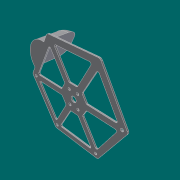
# Autodesk Inventor part: CoilCover
Saved by Autodesk Inventor 2020.4 (Build 244396010, 396A)
## iProperties
Created: 2022-09-10
Part Number: CoilCover
Material: Generic
Document SubType Name: Sheet Metal
Designer: Val
Density: 1 g/cm^3
Sheet Metal Rule: Default
Appearance: Default
Author: Val
Autodesk Inventor part; units mm, degrees
ref_plane "YZ Plane" through (0, 0, 0) normal (1, 0, 0) x (0, 1, 0)
ref_plane "XZ Plane" through (0, 0, 0) normal (0, 1, 0) x (-1, 0, 0)
ref_plane "XY Plane" through (0, 0, 0) normal (0, 0, 1) x (1, 0, 0)
sketch "Base" plane through (0, 0, 0) normal (0, 0, 1) x (1, 0, 0)
  arc A0 (-112.5402, 3.048) -> (-112.5402, -3.048) centre (-107.2609, 0) ccw
  line L0 (-58.9098, 95.9387) -> (-112.5402, 3.048)
  line L1 (-112.5402, -3.048) -> (-58.9098, -95.9387)
  arc A1 (-58.9098, -95.9387) -> (-53.6305, -98.9867) centre (-53.6305, -92.8907) ccw
  arc A2 (53.6305, -98.9867) -> (58.9098, -95.9387) centre (53.6305, -92.8907) ccw
  arc A3 (112.5402, -3.048) -> (112.5402, 3.048) centre (107.2609, 0) ccw
  arc A4 (58.9098, 95.9387) -> (53.6305, 98.9867) centre (53.6305, 92.8907) ccw
  arc A5 (-53.6305, 98.9867) -> (-58.9098, 95.9387) centre (-53.6305, 92.8907) ccw
  line L2 (-53.6305, 98.9867) -> (53.6305, 98.9867)
  line L3 (112.5402, 3.048) -> (58.9098, 95.9387)
  line L4 (58.9098, 95.9387) -> (112.5402, 3.048)
  arc A6 (53.6305, -98.9867) -> (58.9098, -95.9387) centre (53.6305, -92.8907) ccw
  line L5 (112.5402, -3.048) -> (58.9098, -95.9387)
  line L6 (-53.6305, -98.9867) -> (53.6305, -98.9867)
  line L7 (0, 98.9867) -> (0, -98.9867) construction
  line L8 (-113.3569, 0) -> (113.3569, 0) construction
  point P0 (0, 0)
  point P1 (0, 0)
  dimension "d0" = 6.096
  dimension "d1" = 107.2609
  dimension "d2" = 120
  dimension "d3" = 120
  dimension "d4" = 120
  dimension "d5" = 120
  dimension "d6" = 120
  measures "d0" radius of A4
  measures "d1" distance of L2.start L2.end
  measures "d2" angle of L2 L0
  measures "d3" angle of L3 L2
  measures "d4" angle of L6 L1
  measures "d5" angle of L5 L6
  measures "d6" angle of L1 L0
extrude "Plate1" add sketch "Base" along normal blind 3.048
sketch "Cuts" plane through (0, 0, 0) normal (0, 0, -1) x (-1, 0, 0)
  line L0 (0, 0) -> (-56.6785, 98.17) construction
  line L1 (0, 0) -> (-113.3569, 0) construction
  line L2 (0, 0) -> (-56.6785, -98.17) construction
  arc A0 (-53.6305, 98.9867) -> (-58.9098, 95.9387) centre (-53.6305, 92.8907) ccw projected
  arc A1 (-112.5402, 3.048) -> (-112.5402, -3.048) centre (-107.2609, 0) ccw projected
  arc A2 (-58.9098, -95.9387) -> (-53.6305, -98.9867) centre (-53.6305, -92.8907) ccw projected
  line L3 (-112.5402, 3.048) -> (-58.9098, 95.9387) projected
  line L4 (-95.9691, 6.35) -> (-53.4838, 79.9367)
  line L5 (-53.4838, 79.9367) -> (-10.9985, 6.35)
  line L6 (-10.9985, 6.35) -> (-95.9691, 6.35)
  line L7 (-95.9691, -6.35) -> (-53.4838, -79.9367)
  line L8 (-53.4838, -79.9367) -> (-10.9985, -6.35)
  line L9 (-10.9985, -6.35) -> (-95.9691, -6.35)
  line L10 (0, 0) -> (56.6785, 98.17) construction
  arc A3 (58.9098, 95.9387) -> (53.6305, 98.9867) centre (53.6305, 92.8907) ccw projected
  line L11 (0, 0) -> (56.6785, -98.17) construction
  arc A4 (53.6305, -98.9867) -> (58.9098, -95.9387) centre (53.6305, -92.8907) ccw projected
  line L12 (-42.4853, 86.2867) -> (42.4853, 86.2867)
  line L13 (42.4853, 86.2867) -> (0, 12.7)
  line L14 (0, 12.7) -> (-42.4853, 86.2867)
  line L15 (-53.6305, 98.9867) -> (53.6305, 98.9867) projected
  line L16 (-42.4853, -86.2867) -> (42.4853, -86.2867)
  line L17 (42.4853, -86.2867) -> (0, -12.7)
  line L18 (0, -12.7) -> (-42.4853, -86.2867)
  line L19 (0, 0) -> (0, 98.9867) construction
  line L20 (53.6305, 98.9867) -> (-53.6305, 98.9867) projected
  line L21 (95.9691, 6.35) -> (53.4838, 79.9367)
  line L22 (53.4838, 79.9367) -> (10.9985, 6.35)
  line L23 (10.9985, 6.35) -> (95.9691, 6.35)
  line L24 (95.9691, -6.35) -> (53.4838, -79.9367)
  line L25 (53.4838, -79.9367) -> (10.9985, -6.35)
  line L26 (10.9985, -6.35) -> (95.9691, -6.35)
  circle A5 centre (0, 0) radius 6.35
  circle A6 centre (51.5968, 89.3682) radius 3.175
  line L27 (58.9098, 95.9387) -> (112.5402, 3.048) projected
  circle A7 centre (51.5968, 89.3682) radius 9.6185 construction
  arc A8 (112.5402, -3.048) -> (112.5402, 3.048) centre (107.2609, 0) ccw projected
  line L28 (113.3569, 0) -> (0, 0) construction
  circle A9 centre (103.1936, 0) radius 9.6185 construction
  line L29 (112.5402, -3.048) -> (58.9098, -95.9387) projected
  circle A10 centre (103.1936, 0) radius 3.175
  circle A11 centre (51.5968, -89.3682) radius 9.6185 construction
  line L30 (53.6305, -98.9867) -> (-53.6305, -98.9867) projected
  circle A12 centre (51.5968, -89.3682) radius 3.175
  circle A13 centre (-51.5968, 89.3682) radius 3.175
  circle A14 centre (-103.1936, 0) radius 3.175
  circle A15 centre (-51.5968, -89.3682) radius 3.175
  dimension "d12" = 12.7
  dimension "d13" = 6.35
  dimension "d14" = 6.35
  dimension "d15" = 12.7
  dimension "d16" = 6.35
  dimension "d17" = 6.35
  dimension "d21" = 12.7
  dimension "d22" = 6.35
  dimension "d24" = 6.35
  dimension "d25" = 6.35
  constraints: 50 end point, 15 symmetric about line, 8 centre point, 8 point on circle, 5 parallel, 4 coincident, 3 horizontal, 3 point on line, 1 midpoint, 1 tangent, 11 other
  measures "d12" distance between parallel lines of L3 L4
  measures "d13" distance between parallel lines of L0 L5
  measures "d14" distance between parallel lines of L1 L6
  measures "d15" distance between parallel lines of L15 L12
  measures "d16" distance between parallel lines of L0 L14
  measures "d17" distance between parallel lines of L10 L13
  measures "d21" diameter of A5
  measures "d22" diameter of A6
  measures "d24" diameter of A10
  measures "d25" diameter of A12
extrude "CutsFeature" cut sketch "Cuts" against normal blind 3.048 contours L4 L5 L6 | L9 L8 L7 | L12 L13 L14 | L18 L17 L16 | L23 L22 L21 | L24 L25 L26 | A5 | A10 | A12 | A14 | A15
chamfer "Corner Chamfer1" distance 19.05 angle 45 6 edges at (-10.9985, 6.35, 1.524) (0, 12.7, 1.524) (10.9985, 6.35, 1.524) (10.9985, -6.35, 1.524) (0, -12.7, 1.524) (-10.9985, -6.35, 1.524)
fillet "InsideFilletsFeature" radius 3.175 24 edges at (-42.4853, 86.2867, 1.524) (-53.4838, 79.9367, 1.524) (-95.9691, 6.35, 1.524) (42.4853, 86.2867, 1.524) (-53.4838, -79.9367, 1.524) (-95.9691, -6.35, 1.524) (-42.4853, -86.2867, 1.524) (42.4853, -86.2867, 1.524) (53.4838, -79.9367, 1.524) (95.9691, -6.35, 1.524) (95.9691, 6.35, 1.524) (53.4838, 79.9367, 1.524) (30.0485, -6.35, 1.524) (20.5235, -22.8478, 1.524) (30.0485, 6.35, 1.524) (20.5235, 22.8478, 1.524) (9.525, 29.1978, 1.524) (-9.525, 29.1978, 1.524) (-20.5235, 22.8478, 1.524) (-30.0485, 6.35, 1.524) (-30.0485, -6.35, 1.524) (-20.5235, -22.8478, 1.524) (-9.525, -29.1978, 1.524) (9.525, -29.1978, 1.524)
sketch "Sketch4" plane through (0, 0, 0) normal (0, 0, -1) x (-1, 0, 0)
  circle A0 centre (10, 16) radius 3 projected
  circle A1 centre (-10, 16) radius 3 projected
  circle A2 centre (10, -16) radius 3 projected
  circle A3 centre (-10, -16) radius 3 projected
  point P0 (0, 0)
extrude "Cut2" cut sketch "Sketch4" against normal blind 3.048
sketch "Sketch5" plane through (0, 0, 0) normal (0, 0, -1) x (-1, 0, 0)
  circle A0 centre (-10, 16) radius 3 projected
  circle A1 centre (0, 0) radius 18.868 construction
  circle A2 centre (0, 0) radius 11.43 construction
  circle A3 centre (0, 0) radius 25.4 construction
  line L0 (-19.7973, 11.43) -> (-12.0984, 6.985) construction
  line L1 (-21.0673, 9.2303) -> (-13.3684, 4.7853)
  line L2 (-10.8284, 9.1847) -> (-18.5273, 13.6297)
  arc A4 (-18.5273, 13.6297) -> (-21.0673, 9.2303) centre (-19.7973, 11.43) ccw
  arc A5 (-13.3684, 4.7853) -> (-10.8284, 9.1847) centre (-12.0984, 6.985) ccw
  circle A6 centre (0, 0) radius 6.35 construction
  line L3 (-13.97, 2.54) -> (-22.86, 2.54)
  arc A7 (-22.86, 2.54) -> (-22.86, -2.54) centre (-22.86, 0) ccw
  line L4 (-22.86, -2.54) -> (-13.97, -2.54)
  arc A8 (-13.97, -2.54) -> (-13.97, 2.54) centre (-13.97, 0) ccw
  line L5 (-13.3684, -4.7853) -> (-21.0673, -9.2303)
  arc A9 (-21.0673, -9.2303) -> (-18.5273, -13.6297) centre (-19.7973, -11.43) ccw
  line L6 (-18.5273, -13.6297) -> (-10.8284, -9.1847)
  arc A10 (-10.8284, -9.1847) -> (-13.3684, -4.7853) centre (-12.0984, -6.985) ccw
  line L7 (-22.86, 0) -> (0, 0) construction
  line L8 (0.0089, 25.4) -> (0.0089, -25.4) construction
  line L9 (21.0852, 9.2303) -> (13.3862, 4.7853)
  line L10 (10.8462, 9.1847) -> (18.5452, 13.6297)
  arc A11 (21.0852, 9.2303) -> (18.5452, 13.6297) centre (19.8152, 11.43) ccw
  arc A12 (10.8462, 9.1847) -> (13.3862, 4.7853) centre (12.1162, 6.985) ccw
  line L11 (13.9878, 2.54) -> (22.8778, 2.54)
  arc A13 (22.8778, -2.54) -> (22.8778, 2.54) centre (22.8778, 0) ccw
  line L12 (22.8778, -2.54) -> (13.9878, -2.54)
  arc A14 (13.9878, 2.54) -> (13.9878, -2.54) centre (13.9878, 0) ccw
  line L13 (13.3862, -4.7853) -> (21.0852, -9.2303)
  arc A15 (18.5452, -13.6297) -> (21.0852, -9.2303) centre (19.8152, -11.43) ccw
  line L14 (18.5452, -13.6297) -> (10.8462, -9.1847)
  arc A16 (13.3862, -4.7853) -> (10.8462, -9.1847) centre (12.1162, -6.985) ccw
  point P0 (-15.9479, 9.2075)
  dimension "d31" = 5.08
  dimension "d32" = 5.08
  dimension "d33" = 50.8
  dimension "d36" = 60
  constraints: 32 end point, 26 point on circle, 18 symmetric about line, 14 centre point, 6 tangent, 3 coincident, 1 horizontal, 1 midpoint, 1 parallel, 1 point on line, 1 vertical, 30 other
  measures "d31" diameter of A5
  measures "d32" radial gap between concentric circles of A6 A2
  measures "d33" diameter of A3
cut "Cut3" [suppressed]
equation "\"d3\" = d2"
equation "\"d4\" = d2"
equation "\"d5\" = d2"
equation "\"d6\" = d2"
equation "\"d15\" = d12"
equation "\"d16\" = d13"
equation "\"d17\" = d13"
equation "\"d18\" = Thickness"
equation "\"d29\" = Thickness"
equation "\"d38\" = Thickness"
equation "\"d11\" = Thickness"
equation "\"BendRadius\" = Thickness"
equation "\"BendReliefWidth\" = Thickness"
equation "\"BendReliefDepth\" = 0.5 * Thickness"
equation "\"CornerReliefSize\" = 4 * Thickness"
equation "\"MinimumRemnant\" = 2 * Thickness"
equation "\"TransitionRadius\" = BendRadius"
equation "\"JacobiRadiusSize\" = BendRadius"
equation "\"GapSize\" = Thickness"
equation "\"Thickness\" = 3.048"
body "Solid1"
